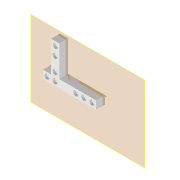
# Autodesk Inventor part: 30_Scanlens_Laseradaper_lid_v1
Saved by Autodesk Inventor 2022 (Build 260153000, 153)
## iProperties
Created: 2022-12-18
Part Number: 30_Scanlens_Laseradaper_lid_v1
Material: Generisch
Document SubType Name: Modeling
Designer: diederichbenedict
Density: 1 g/cm^3
Appearance: Vorgabe
Author: diederichbenedict
Autodesk Inventor part; units mm, degrees
ref_plane "YZ Plane" through (0, 0, 0) normal (1, 0, 0) x (0, 1, 0)
ref_plane "XZ Plane" through (0, 0, 0) normal (0, 1, 0) x (-1, 0, 0)
ref_plane "XY Plane" through (0, 0, 0) normal (0, 0, 1) x (1, 0, 0)
ref_plane "Arbeitsebene1" through (9.85, -10, -4.9007) normal (0, -1, 0) x (-1, 0, 0)
sketch "Skizze1" plane through (9.85, -10, -4.9007) normal (0, -1, 0) x (-1, 0, 0)
  circle A0 centre (3.75, -4.8993) radius 7 projected
  line L0 (22.75, 4.9007) -> (-22.75, 4.9007) projected
  line L1 (-22.75, 4.9007) -> (-22.75, -4.9007) projected
  line L2 (-22.75, -4.9007) -> (-2.35, -4.9007) projected
  arc A1 (9.85, -4.9007) -> (-2.35, -4.9007) centre (3.75, -4.8993) ccw projected
  line L3 (9.85, -4.9007) -> (22.75, -4.9007) projected
  line L4 (22.75, -4.9007) -> (22.75, 4.9007) projected
  circle A2 centre (3.75, -4.8993) radius 6.1 projected
  line L5 (-17.6699, -15.6993) -> (-22.75, -15.6993) projected
  line L6 (22.75, -4.9007) -> (-22.75, -4.9007)
  line L7 (-22.75, -4.9007) -> (-22.75, -15.6993)
  line L8 (-22.75, -15.6993) -> (22.75, -15.6993)
  line L9 (22.75, -15.6993) -> (22.75, -4.9007)
  point P0 (-22.75, -4.9007)
  point P1 (-17.6699, -15.6993)
  point P2 (10.75, -4.9007)
  point P3 (-3.25, -4.9007)
  constraints: 8 end point, 2 parallel, 1 horizontal, 1 perpendicular
ref_plane "Arbeitsebene2" through (-2.9, 0, -9.8015) normal (0, 1, 0) x (0, 0, 1)
extrude "Extrusion1" add sketch "Skizze1" against normal up to surface (10 mm away) contours L3 L9 L8 L5 L7 L2 A0 | A0 L2 A2 L3
sketch "Skizze2" plane through (-12.9, -10, 10.7985) normal (0, 0, 1) x (1, 0, 0)
  circle A0 centre (5, 5) radius 1.4 projected
  circle A1 centre (30.5801, 5) radius 1.4 projected
  circle A2 centre (40.4199, 5) radius 1.4 projected
  point P0 (12.9, 10)
hole "Bohrung1" at (-7.9, -5, 10.7985) at (17.6801, -5, 10.7985) at (27.5199, -5, 10.7985) direction (0, 0, -1) diameter 2.9 end through all counterbore diameter 6.5 counterbore depth 3
sketch "Skizze3" plane through (-12.9, -10, 10.7985) normal (0, 0, 1) x (1, 0, 0)
  circle A0 centre (30.5801, 5) radius 3.25 projected
  circle A1 centre (5, 5) radius 3.25 projected
  circle A2 centre (40.4199, 5) radius 3.25 projected
  line L0 (45.5, 10) -> (0, 10) projected
  line L1 (0, 0) -> (0, 10) projected
  line L2 (45.5, 0) -> (0, 0) projected
  line L3 (45.5, 0) -> (45.5, 10) projected
  line L4 (10, 18) -> (10, 10.0274) projected
  line L5 (3, 32.1736) -> (3, 14.9264) projected
  arc A3 (7, 32.1736) -> (3, 32.1736) centre (5, 32.1736) ccw projected
  line L6 (7, 14.9264) -> (7, 32.1736) projected
  arc A4 (3, 14.9264) -> (7, 14.9264) centre (5, 14.9264) ccw projected
  line L7 (12, 32.1736) -> (12, 20) projected
  arc A5 (12, 32.1736) -> (11.6196, 34.4497) centre (5, 32.1736) ccw projected
  arc A6 (13.5109, 37.1) -> (11.6196, 34.4497) centre (13.5109, 35.1) ccw projected
  line L8 (0.027, 37.1) -> (13.5109, 37.1) projected
  arc A7 (0.027, 37.1) -> (0, 37.0726) centre (5, 32.1736) ccw projected
  line L9 (0, 10.0274) -> (0, 37.0726) projected
  arc A8 (0, 10.0274) -> (0.027, 10) centre (5, 14.9264) ccw projected
  line L10 (9.973, 10) -> (0.027, 10) projected
  arc A9 (9.973, 10) -> (10, 10.0274) centre (5, 14.9264) ccw projected
  line L11 (10, 18) -> (10, 10.0274) projected
  arc A10 (12, 20) -> (10, 18) centre (12, 18) ccw projected
  line L12 (0, 10) -> (12.9, 10) projected
  line L13 (0, 10) -> (10, 10)
  line L14 (10, 10) -> (10, 48)
  line L15 (10, 48) -> (0, 48)
  line L16 (0, 48) -> (0, 10)
  line L17 (45.5, 0) -> (0, 0) projected
  line L18 (45.5, 0) -> (55.5, 0)
  line L19 (55.5, 0) -> (55.5, 10)
  line L20 (55.5, 10) -> (45.5, 10)
  line L21 (45.5, 10) -> (45.5, 0)
  line L22 (0, 0) -> (0, 10) projected
  line L23 (0, 0) -> (-10, 0)
  line L24 (-10, 0) -> (-10, 10)
  line L25 (-10, 10) -> (0, 10)
  line L26 (0, 10) -> (0, 0)
  point P0 (0, 10)
  point P1 (45.5, 10)
  point P2 (0, 37.0726)
  dimension "d9" = 38
  dimension "d10" = 10
  dimension "d11" = 10
  dimension "d12" = 10
  dimension "d13" = 10
  constraints: 24 end point, 6 parallel, 3 horizontal, 3 perpendicular
  measures "d9" distance of L14.end L13.end
  measures "d10" distance of L20.end L19.end
  measures "d11" distance of L19.end L18.end
  measures "d12" distance of L24.end L25.end
  measures "d13" distance of L23.end L24.end
ref_plane "Arbeitsebene4" through (-15.175, -1.3586, -0.0015) normal (0, 0, -1) x (0, 1, 0)
extrude "Extrusion2" add sketch "Skizze3" against normal up to surface (10.8 mm away) contours L20 L19 L18 L3 | L23 L24 L25 L1 | L0 A8 L9 A7 L8 L14 L4 A9 | L8 A7 L16 L15 L14 | A3 L6 A4 L5
sketch "Skizze4" plane through (-22.9, -10, 10.7985) normal (0, 0, 1) x (1, 0, 0)
  circle A0 centre (40.5801, 5) radius 3.25 projected
  circle A1 centre (15, 5) radius 3.25 projected
  circle A2 centre (50.4199, 5) radius 3.25 projected
  line L0 (65.5, 10) -> (19.973, 10) projected
  arc A3 (19.973, 10) -> (20, 10.0274) centre (15, 14.9264) ccw projected
  line L1 (20, 10.0274) -> (20, 48) projected
  line L2 (20, 48) -> (10, 48) projected
  line L3 (10, 48) -> (10, 10.0274) projected
  arc A4 (10, 10.0274) -> (10.027, 10) centre (15, 14.9264) ccw projected
  line L4 (10.027, 10) -> (0, 10) projected
  line L5 (0, 10) -> (0, 0) projected
  line L6 (65.5, 0) -> (0, 0) projected
  line L7 (65.5, 0) -> (65.5, 10) projected
  circle A5 centre (60.5, 5) radius 1.4
  circle A6 centre (15.4264, 43) radius 1.4
  circle A7 centre (5, 5) radius 1.4
  circle A8 centre (15, 32.1736) radius 1.4
  line L8 (13, 32.1736) -> (13, 14.9264) projected
  line L9 (17, 14.9264) -> (17, 32.1736) projected
  arc A9 (13, 14.9264) -> (17, 14.9264) centre (15, 14.9264) ccw projected
  arc A10 (17, 32.1736) -> (13, 32.1736) centre (15, 32.1736) ccw projected
  point P0 (22.9, 10)
  dimension "d16" = 2.8
  dimension "d17" = 2.8
  dimension "d18" = 2.8
  dimension "d19" = 5
  dimension "d20" = 5
  dimension "d21" = 5
  dimension "d29" = 2.8
  constraints: 4 centre point, 1 coincident
  measures "d16" diameter of A5
  measures "d17" diameter of A6
  measures "d18" diameter of A7
  measures "d19" distance from line of A5.centre L7
  measures "d20" distance from line of A6.centre L2
  measures "d21" distance from line of L5 A7.centre
  measures "d29" diameter of A8
hole "Bohrung2" at (37.6, -5, 10.7985) at (-17.9, -5, 10.7985) at (-7.4736, 33, 10.7985) at (-7.9, 22.1736, 10.7985) at (-7.9, 4.9264, 10.7985) direction (0, 0, -1) diameter 2.9 end through all counterbore diameter 6.5 counterbore depth 3
ref_plane "Arbeitsebene3" through (24.5, -13.25, 2.8735) normal (0, 0, 1) x (-1, 0, 0)
